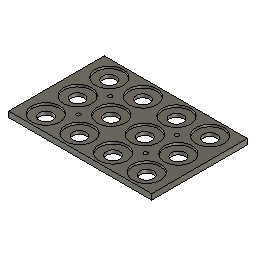
20cc_vial_plate_retainerlid v2 (Autodesk Fusion 360 design; units mm, degrees)
Autodesk Fusion 360 part; units mm, degrees
sketch "Sketch1" plane through (0, 0, 0) normal (0, 0, 1) x (1, 0, 0)
  line L0 (0, 0) -> (127.76, 0)
  line L1 (127.76, 0) -> (127.76, -85.48)
  line L2 (127.76, -85.48) -> (0, -85.48)
  line L3 (0, -85.48) -> (0, 0)
  dimension "d1" = 127.76
  dimension "d2" = 85.48
  constraint horizontal L0
  constraint vertical L1
  constraint horizontal L2
  constraint vertical L3
  constraint coincident L0.start L3.end
  measures "d1" distance of L0.start L0.end
  measures "d2" distance of L0.start L2.end
extrude "Extrude1" add sketch "Sketch1" along normal blind 5
sketch "Sketch7" plane through (0, 0, 5) normal (0, 0, 1) x (-1, 0, 0)
  line L0 (0, 85.48) -> (-127.76, 85.48)
  line L1 (-127.76, 85.48) -> (-127.76, 0)
  line L2 (-127.76, 0) -> (0, 0)
  line L3 (0, 0) -> (0, 85.48)
  point P0 (-18.875, 14.4325)
  point P1 (-48.878, 14.4325)
  point P2 (-78.881, 14.4325)
  point P3 (-108.884, 14.4325)
  point P4 (-18.875, 42.74)
  point P5 (-48.878, 42.74)
  point P6 (-78.881, 42.74)
  point P7 (-108.884, 42.74)
  point P8 (-18.875, 71.0475)
  point P9 (-48.878, 71.0475)
  point P10 (-78.881, 71.0475)
  point P11 (-108.884, 71.0475)
  dimension "d42" = -30.003
  dimension "d43" = 28.3075
hole "Hole1" at (18.875, -14.4325, 5) at (18.875, -42.74, 5) at (18.875, -71.0475, 5) at (48.878, -71.0475, 5) at (48.878, -42.74, 5) at (48.878, -14.4325, 5) at (78.881, -14.4325, 5) at (78.881, -42.74, 5) at (78.881, -71.0475, 5) at (108.884, -71.0475, 5) at (108.884, -42.74, 5) at (108.884, -14.4325, 5) direction (0, 0, -1) diameter 12 depth 13 tip angle 180 counterbore diameter 24.8 counterbore depth 2
sketch "Sketch8" plane through (0, 0, 0) normal (0, 0, -1) x (1, 0, 0)
  circle A0 centre (108.884, 42.74) radius 6
  circle A1 centre (78.881, 71.0475) radius 6
  circle A2 centre (78.881, 14.4325) radius 6
  circle A3 centre (48.878, 42.74) radius 6
  circle A4 centre (18.875, 71.0475) radius 6
  circle A5 centre (18.875, 14.4325) radius 6
  circle A6 centre (18.875, 42.74) radius 6
  circle A7 centre (48.878, 71.0475) radius 6
  circle A8 centre (48.878, 14.4325) radius 6
  circle A9 centre (78.881, 42.74) radius 6
  circle A10 centre (108.884, 71.0475) radius 6
  circle A11 centre (108.884, 14.4325) radius 6
  line L0 (127.76, 85.48) -> (0, 85.48)
  line L1 (0, 85.48) -> (0, 0)
  line L2 (0, 0) -> (127.76, 0)
  line L3 (127.76, 0) -> (127.76, 85.48)
  point P0 (33.877, 28.587)
  point P1 (93.883, 28.587)
  point P2 (33.877, 56.8945)
  point P3 (93.883, 56.8945)
  dimension "d52" = 60.006
  dimension "d53" = 28.3075
hole "Hole3" at (33.877, -56.8945, 0) at (33.877, -28.587, 0) at (93.883, -56.8945, 0) at (93.883, -28.587, 0) direction (0, 0, 1) diameter 3.4 depth 20 tip angle 118 counterbore diameter 6 counterbore depth 2.5
